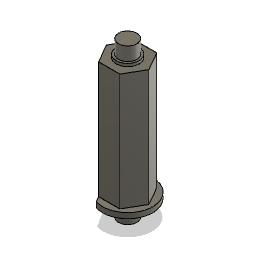
Axle (Autodesk Fusion 360 design; units mm, degrees)
Autodesk Fusion 360 part; units mm, degrees
sketch "Sketch1" plane through (0, 0, 0) normal (0, 1, 0) x (1, 0, 0)
  circle A0 centre (0, 0) radius 3.125
  circle A1 centre (0, 0) radius 3.887
  line L0 (7.2169, 0) -> (3.6084, 6.25)
  line L1 (3.6084, 6.25) -> (-3.6084, 6.25)
  line L2 (-3.6084, 6.25) -> (-7.2169, 0)
  line L3 (-7.2169, 0) -> (-3.6084, -6.25)
  line L4 (-3.6084, -6.25) -> (3.6084, -6.25)
  line L5 (3.6084, -6.25) -> (7.2169, 0)
  line L6 (-8.2931, 1.8641) -> (-2.5322, -8.1141)
  arc A2 (-2.5322, -8.1141) -> (-8.2931, 1.8641) centre (0, 0) ccw
  dimension "d1" = 6.25
  dimension "d2" = 0.762
  dimension "d3" = 6.25
  dimension "d22" = 8.5
  constraint coincident A0.centre A1.centre
  constraint horizontal L1
  constraint collinear L3 L6
  measures "d1" diameter of A0
  measures "d2" distance of A0 A1
  measures "d3" distance of A0.centre L5
  measures "d22" radius of A2
extrude "Extrude1" add sketch "Sketch1" along normal blind 4.572 contours A0
extrude "Extrude2" add sketch "Sketch1" along normal blind 0.9652 from surface at 4.572 contours A0 | A1
extrude "Extrude3" add sketch "Sketch1" along normal blind 41.402 from surface at 5.5372 contours A0 | A1 | L0 L1 L2 L3 L4 L5 L6
extrude "Extrude4" add sketch "Sketch1" along normal blind 0.9652 from surface at 46.9392 contours A0 | A1
extrude "Extrude5" add sketch "Sketch1" along normal blind 4.572 from surface at 47.9044 contours A0
extrude "Extrude6" add sketch "Sketch1" along normal blind 1.8 from surface at 5.5372 contours L0 L1 L2 L4 L5 L6 A2
equation "d1 = ( ( 1 / 4 ) * 1 ) * 1 in - 0.1 mm"
equation "d3 = 0.25 in - 0.1 mm"
